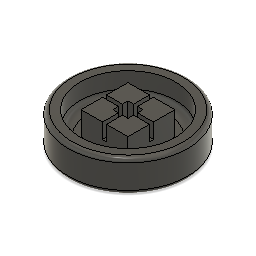
DC801-BM-Joy-Hats v29 (Autodesk Fusion 360 design; units mm, degrees)
Autodesk Fusion 360 part; units mm, degrees
note: some values were not read from the file. Chosen so that the rebuilt part matches the saved one: which face or edge a step refers to. Set by a fixed rule: which sketch regions a step uses.
sketch "Sketch1" plane through (0, 0, 0) normal (0, 1, 0) x (1, 0, 0)
  line L0 (0.95, 0.95) -> (-0.95, 0.95)
  line L1 (-0.95, 0.95) -> (-0.95, -0.95)
  line L2 (-0.95, -0.95) -> (0.95, -0.95)
  line L3 (0.95, -0.95) -> (0.95, 0.95)
  line L4 (0.95, 0.95) -> (-0.95, -0.95) construction
  line L5 (-0.95, 0.95) -> (0.95, -0.95) construction
  circle A0 centre (0, 0) radius 7.5
  line L6 (0.25, -2.95) -> (-0.25, -2.95)
  line L7 (-0.25, -2.95) -> (-0.25, 2.95)
  line L8 (-0.25, 2.95) -> (0.25, 2.95)
  line L9 (0.25, 2.95) -> (0.25, -2.95)
  line L10 (0.25, -2.95) -> (-0.25, 2.95) construction
  line L11 (-0.25, -2.95) -> (0.25, 2.95) construction
  line L12 (2.95, 2.95) -> (-2.95, 2.95)
  line L13 (-2.95, 2.95) -> (-2.95, -2.95)
  line L14 (-2.95, -2.95) -> (2.95, -2.95)
  line L15 (2.95, -2.95) -> (2.95, 2.95)
  circle A1 centre (0, 0) radius 6
  line L16 (2.95, 0.25) -> (-2.95, 0.25)
  line L17 (-2.95, 0.25) -> (-2.95, -0.25)
  line L18 (-2.95, -0.25) -> (2.95, -0.25)
  line L19 (2.95, -0.25) -> (2.95, 0.25)
  line L20 (2.95, 0.25) -> (-2.95, -0.25) construction
  line L21 (-2.95, 0.25) -> (2.95, -0.25) construction
  dimension "d1" = 1.9
  dimension "d2" = 1.9
  dimension "d3" = 15
  dimension "d35" = 0.5
  dimension "d63" = 2
  dimension "d68" = 2
  dimension "d71" = 0.5
  dimension "d94" = 5.9
  dimension "d96" = 5.9
  constraint horizontal L0
  constraint perpendicular L0 L1
  constraint parallel L0 L2
  constraint parallel L1 L3
  constraint coincident L4 A0.centre
  constraint coincident L5 A0.centre
  constraint coincident A0.centre A1.centre
  constraint horizontal L6
  constraint perpendicular L6 L7
  constraint parallel L6 L8
  constraint parallel L7 L9
  constraint coincident L10 A0.centre
  constraint coincident L11 A0.centre
  constraint horizontal L16
  constraint perpendicular L16 L17
  constraint parallel L16 L18
  constraint parallel L17 L19
  constraint coincident L20 A0.centre
  constraint coincident L21 A0.centre
  measures "d1" distance of L1.end L2.end
  measures "d2" distance of L0.end L1.end
  measures "d3" diameter of A0
  measures "d35" distance of L7.end L8.end
  measures "d63" distance of L2 L6
  measures "d71" distance of L16.end L17.end
  measures "d94" distance of L16.start L16.end
  measures "d96" distance of L6.start L8.end
extrude "Extrude1" add sketch "Sketch1" along normal blind 3 contours L0 L3 L9 L12 L15 L16 | L0 L1 L7 L12 L13 L16 | L2 L3 L9 L14 L15 L18 | L1 L2 L7 L13 L14 L18 | A0 makes body 1 at (2.95, 1, -1.15) makes body 2 at (2.95, 1, 2.05) makes body 3 at (-1.15, 1, -2.95) makes body 4 at (7.4907, 2, 0.3738) makes body 5 at (-2.95, 1, 1.15)
extrude "Extrude12" add sketch "Sketch1" against normal blind 1 contours L0 L3 L9 L16 | L0 L3 L9 L12 L15 L16 | L0 L7 L9 L16 | L0 L7 L8 L9 L12 | L3 L15 L16 L18 L19 | L3 L9 L16 L18 | L0 L1 L7 L16 | L0 L1 L7 L12 L13 L16 | L7 L9 L16 L18 | L2 L3 L9 L14 L15 L18 | L2 L3 L9 L18 | L1 L7 L16 L18 | L2 L7 L9 L18 | L1 L13 L16 L17 L18 | L1 L2 L7 L18 | L2 L6 L7 L9 L14 | L1 L2 L7 L13 L14 L18 | A0 | A1 bodies 1 2 3 4 5
sketch "Sketch17" plane through (0, 0, 0) normal (0, 1, 0) x (-1, 0, 0)
  line L0 (-2.95, -2.95) -> (-2.95, -0.25)
  line L1 (-2.95, -0.25) -> (-0.95, -0.25)
  line L2 (-0.95, -0.25) -> (-0.95, -0.95)
  line L3 (-0.95, -0.95) -> (-0.25, -0.95)
  line L4 (-0.25, -0.95) -> (-0.25, -2.95)
  line L5 (-0.25, -2.95) -> (-2.95, -2.95)
  line L6 (2.95, -2.95) -> (0.25, -2.95)
  line L7 (0.25, -2.95) -> (0.25, -0.95)
  line L8 (0.25, -0.95) -> (0.95, -0.95)
  line L9 (0.95, -0.95) -> (0.95, -0.25)
  line L10 (0.95, -0.25) -> (2.95, -0.25)
  line L11 (2.95, -0.25) -> (2.95, -2.95)
  line L12 (2.95, 2.95) -> (2.95, 0.25)
  line L13 (2.95, 0.25) -> (0.95, 0.25)
  line L14 (0.95, 0.25) -> (0.95, 0.95)
  line L15 (0.95, 0.95) -> (0.25, 0.95)
  line L16 (0.25, 0.95) -> (0.25, 2.95)
  line L17 (0.25, 2.95) -> (2.95, 2.95)
  line L18 (-2.95, 2.95) -> (-0.25, 2.95)
  line L19 (-0.25, 2.95) -> (-0.25, 0.95)
  line L20 (-0.25, 0.95) -> (-0.95, 0.95)
  line L21 (-0.95, 0.95) -> (-0.95, 0.25)
  line L22 (-0.95, 0.25) -> (-2.95, 0.25)
  line L23 (-2.95, 0.25) -> (-2.95, 2.95)
  line L24 (-2.95, -2.95) -> (2.95, -2.95)
  line L25 (2.95, -2.95) -> (2.95, 2.95)
  line L26 (2.95, 2.95) -> (-2.95, 2.95)
  line L27 (-2.95, 2.95) -> (-2.95, -2.95)
  line L28 (-2.95, -2.95) -> (2.95, 2.95) construction
  line L29 (2.95, -2.95) -> (-2.95, 2.95) construction
  circle A0 centre (0, 0) radius 6
  dimension "d103" = 5.9
  dimension "d104" = 5.9
  constraint horizontal L24
  constraint perpendicular L24 L25
  constraint parallel L24 L26
  constraint parallel L25 L27
  constraint coincident L28 A0.centre
  constraint coincident L29 A0.centre
  measures "d103" distance of L12.start L18.start
  measures "d104" distance of L6.start L12.start
extrude "Extrude18" add sketch "Sketch17" along normal blind 1.1 contours L1 L2 L3 L4 L7 L8 L9 L10 L13 L14 L15 L16 L19 L20 L21 L22 L24 L25 L26 L27 bodies 1
fillet "Fillet6" radius 0.5 2 edges at (-6.9925, 3, 2.7121) (-6.9925, -1, -2.7121) on bodies 1
fillet "Fillet7" radius 1 1 edges at (-5.594, 0, -2.1697) on bodies 1
